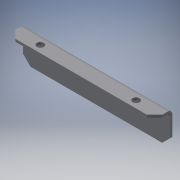
# Autodesk Inventor part: Part103
Saved by Autodesk Inventor 2016 (Build 200138000, 138)
## iProperties
Created: 2018-11-13
Part Number: Part103
Material: Generic
Document SubType Name: Sheet Metal
Designer: hovm
Density: 1 g/cm^3
Sheet Metal Rule: Default_mm
Appearance: Default
Author: hovm
Autodesk Inventor part; units mm, degrees
ref_plane "YZ Plane" through (0, 0, 0) normal (1, 0, 0) x (0, 1, 0)
ref_plane "XZ Plane" through (0, 0, 0) normal (0, 1, 0) x (-1, 0, 0)
ref_plane "XY Plane" through (0, 0, 0) normal (0, 0, 1) x (1, 0, 0)
sketch "Sketch1" plane through (0, 0, 0) normal (0, 0, 1) x (1, 0, 0)
  line L0 (-57.5, -7) -> (57.5, -7)
  line L1 (57.5, -7) -> (57.5, 7)
  line L2 (57.5, 7) -> (-57.5, 7)
  line L3 (-57.5, 7) -> (-57.5, -7)
  line L4 (-57.5, -7) -> (57.5, 7) construction
  line L5 (57.5, -7) -> (-57.5, 7) construction
  point P0 (0, 0)
  dimension "d0" = 115
  dimension "d1" = 14
  measures "d0" distance of L1.end L2.end
  measures "d1" distance of L0.end L1.end
extrude "Plate1" add sketch "Sketch1" along normal blind 2
sketch "Sketch2" plane through (57.5, 5, 2) normal (0, 1, 0) x (-1, 0, 0)
  line L0 (115, 0) -> (0, 0)
  line L1 (0, 0) -> (0, -25)
  line L2 (0, -25) -> (115, -25)
  line L3 (115, -25) -> (115, 0)
  constraints: 6 end point, 1 horizontal, 1 perpendicular, 1 vertical
edge flange "Flange1" height 25 angle 90 thickness 2 bend radius 2 thickness toward (0, 1, 0) relief tear relief width 2 relief depth 1 edges at (0, 7, 0) wall of the first edge with corners at (-57.5, 5, 2) (57.5, 5, 2) (57.5, 5, -23) (-57.5, 5, -23)
bend "Bend1"
corner "Corner1"
chamfer "Corner Chamfer1" distance 6 angle 45 4 edges at (-57.5, -7, 1) (57.5, -7, 1) (-57.5, 6, -23) (57.5, 6, -23)
sketch "Sketch3" plane through (0, 0, 2) normal (0, 0, 1) x (1, 0, 0)
  circle A0 centre (-37.5, -132.5) radius 2.9585 projected
  circle A1 centre (37.5, -132.5) radius 2.9585 projected
  circle A2 centre (-5, -1.3494) radius 3.1 projected
  point P0 (0, 0)
  point P1 (-37.5, -1.3494)
  point P2 (37.5, -1.3494)
  constraints: 2 horizontal alignment, 2 vertical alignment
hole "Hole1" at (-37.5, -1.3494, 2) at (37.5, -1.3494, 2) direction (0, 0, -1) diameter 5.5 depth 2 tip angle 118
sketch "Sketch4" plane through (0, 0, 0) normal (0, 0, -1) x (-1, 0, 0)
  point P0 (0, 0)
equation "\"d21\" = Thickness"
equation "\"d3\" = BendReliefWidth"
equation "\"d4\" = BendReliefDepth"
equation "\"d5\" = MinimumRemnant"
equation "\"d6\" = BendRadius"
equation "\"d9\" = BendRadius"
equation "\"d10\" = CornerReliefSize"
equation "\"d11\" = GapSize"
equation "\"d12\" = JacobiRadiusSize"
equation "\"BendRadius\" = Thickness"
equation "\"BendReliefWidth\" = Thickness"
equation "\"BendReliefDepth\" = 0.5 * Thickness"
equation "\"CornerReliefSize\" = 4 * Thickness"
equation "\"MinimumRemnant\" = 2 * Thickness"
equation "\"TransitionRadius\" = BendRadius"
equation "\"JacobiRadiusSize\" = BendRadius"
equation "\"GapSize\" = Thickness"
equation "\"d2\" = BendRadius"
equation "\"Thickness\" = 2"
body "Solid1"
